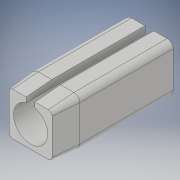
# Autodesk Inventor part: hjul-motor overgang
Saved by Autodesk Inventor 2019 (Build 230136000, 136)
## iProperties
Created: 2019-03-12
Part Number: hjul-motor overgang
Material: Generic
Document SubType Name: Modeling
Designer: jonas
Density: 1 g/cm^3
Appearance: Default
Author: jonas
Autodesk Inventor part; units mm, degrees
ref_plane "YZ Plane" through (0, 0, 0) normal (1, 0, 0) x (0, 1, 0)
ref_plane "XZ Plane" through (0, 0, 0) normal (0, 1, 0) x (-1, 0, 0)
ref_plane "XY Plane" through (0, 0, 0) normal (0, 0, 1) x (1, 0, 0)
sketch "Sketch1" plane through (0, 0, 0) normal (0, 0, 1) x (1, 0, 0)
  line L0 (-1.2, 1.6) -> (-0.2919, 1.6)
  line L1 (1.6, 1.2) -> (1.6, -1.2)
  line L2 (1.2, -1.6) -> (-1.2, -1.6)
  line L3 (-1.6, -1.2) -> (-1.6, 1.2)
  line L4 (0, -2.356) -> (0, 2.356) projected
  line L5 (-2.356, 0) -> (2.356, 0) projected
  arc A0 (-0.2919, 1.1123) -> (0.2919, 1.1123) centre (0, 0) ccw
  line L6 (0.2919, 1.6) -> (0.2919, 1.1123)
  line L7 (0.2919, 1.6) -> (1.2, 1.6)
  line L8 (-0.2919, 1.1123) -> (-0.2919, 1.6)
  arc A1 (1.6, 1.2) -> (1.2, 1.6) centre (1.2, 1.2) ccw
  arc A2 (1.2, -1.6) -> (1.6, -1.2) centre (1.2, -1.2) ccw
  arc A3 (-1.6, -1.2) -> (-1.2, -1.6) centre (-1.2, -1.2) ccw
  arc A4 (-1.2, 1.6) -> (-1.6, 1.2) centre (-1.2, 1.2) ccw
  dimension "d0" = 1.6
  dimension "d2" = 2.3
  dimension "d6" = 0.4
  constraints: 14 end point, 10 point on circle, 8 tangent, 5 centre point, 4 parallel, 3 equal radius, 2 horizontal, 2 perpendicular, 1 coincident, 2 other
  measures "d0" distance between parallel lines of L1 L4
  measures "d2" diameter of A0
  measures "d6" radius of A1
extrude "Extrusion2" add sketch "Sketch1" along normal blind 8 contours L0 L8 A0 L5 L3 A4 | L5 A0 L4 L2 A3 L3 | A0 L5 L1 A2 L2 L4 | A0 L6 L7 A1 L1 L5
chamfer "Chamfer1" distance 0.15 angle 85 9 edges at (1.6, 0, 8) (1.4828, 1.4828, 8) (0.746, 1.6, 8) (1.4828, -1.4828, 8) (0, -1.6, 8) (-1.4828, -1.4828, 8) (-1.6, 0, 8) (-1.4828, 1.4828, 8) (-0.746, 1.6, 8) measured on face at (-1.4476, 0.0429, 8)
equation "\"d0\" = d1"
equation "\"d1\" = 1.6"
body "Solid2"
